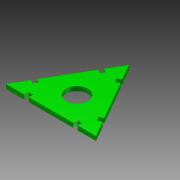
# Autodesk Inventor part: actuator
Saved by Autodesk Inventor 2012 (Build 160160000, 160)
## iProperties
Created: 2013-10-02
Part Number: actuator
Material: Default
Document SubType Name: Modeling
Designer: Nick
Density: 1 g/cm^3
Author: Nick
Autodesk Inventor part; units mm, degrees
ref_plane "YZ Plane" through (0, 0, 0) normal (1, 0, 0) x (0, 1, 0)
ref_plane "XZ Plane" through (0, 0, 0) normal (0, 1, 0) x (-1, 0, 0)
ref_plane "XY Plane" through (0, 0, 0) normal (0, 0, 1) x (1, 0, 0)
sketch "Sketch1" plane through (0, 0, 0) normal (0, 0, 1) x (1, 0, 0)
  circle A0 centre (0, 0) radius 7.5
  line L0 (31.1769, -18) -> (-31.1769, -18) construction
  line L1 (-31.1769, -18) -> (0, 36) construction
  line L2 (0, 36) -> (31.1769, -18) construction
  line L3 (15.5, -18) -> (15.5, -15)
  line L4 (15.5, -15) -> (18.5, -15)
  line L5 (18.5, -15) -> (18.5, -18)
  line L6 (-18.5, -18) -> (-18.5, -15)
  line L7 (-18.5, -15) -> (-15.5, -15)
  line L8 (-15.5, -15) -> (-15.5, -18)
  line L9 (-31.1769, -18) -> (15.5885, 9) construction
  line L10 (31.1769, -18) -> (-15.5885, 9) construction
  line L11 (0, 36) -> (0, -18) construction
  line L12 (6.3385, 25.0215) -> (3.7404, 23.5215)
  line L13 (3.7404, 23.5215) -> (5.2404, 20.9234)
  line L14 (5.2404, 20.9234) -> (7.8385, 22.4234)
  line L15 (23.3385, -4.4234) -> (20.7404, -5.9234)
  line L16 (20.7404, -5.9234) -> (22.2404, -8.5215)
  line L17 (22.2404, -8.5215) -> (24.8385, -7.0215)
  line L18 (-24.8385, -7.0215) -> (-22.2404, -8.5215)
  line L19 (-22.2404, -8.5215) -> (-20.7404, -5.9234)
  line L20 (-20.7404, -5.9234) -> (-23.3385, -4.4234)
  line L21 (-7.8385, 22.4234) -> (-5.2404, 20.9234)
  line L22 (-5.2404, 20.9234) -> (-3.7404, 23.5215)
  line L23 (-3.7404, 23.5215) -> (-6.3385, 25.0215)
  line L24 (-6.3385, 25.0215) -> (0, 36)
  line L25 (6.3385, 25.0215) -> (0, 36)
  line L26 (7.8385, 22.4234) -> (23.3385, -4.4234)
  line L27 (24.8385, -7.0215) -> (31.1769, -18)
  line L28 (31.1769, -18) -> (18.5, -18)
  line L29 (15.5, -18) -> (-15.5, -18)
  line L30 (-18.5, -18) -> (-31.1769, -18)
  line L31 (-31.1769, -18) -> (-24.8385, -7.0215)
  line L32 (-23.3385, -4.4234) -> (-7.8385, 22.4234)
  dimension "d3" = 15
  dimension "d4" = 18.5
  dimension "d5" = 18.5
  dimension "d8" = 3
  dimension "d9" = 18
  dimension "d10" = 3
  dimension "d11" = 3
  dimension "d12" = 18.5
  dimension "d13" = 3
  dimension "d14" = 3
  dimension "d15" = 18.5
  dimension "d16" = 3
  dimension "d17" = 3
  dimension "d18" = 18.5
  dimension "d19" = 3
  dimension "d20" = 3
  dimension "d21" = 3
  dimension "d22" = 18.5
  dimension "d23" = 3
  constraints: 66 end point, 14 perpendicular, 12 point on line, 7 collinear, 6 parallel, 3 midpoint, 2 coincident, 1 centre point, 1 horizontal, 7 other
  measures "d3" diameter of A0
  measures "d4" distance from line of L5 A0.centre
  measures "d5" horizontal distance of point (0, 0) L6.start
  measures "d8" distance between parallel lines of L0 L4
  measures "d9" distance from line of L0 point (0, 0)
  measures "d10" distance between parallel lines of L5 L3
  measures "d11" distance between parallel lines of L6 L8
  measures "d12" distance between parallel lines of L17 L9
  measures "d13" distance between parallel lines of L15 L17
  measures "d14" distance between parallel lines of L2 L16
  measures "d15" distance between parallel lines of L12 L9
  measures "d16" distance between parallel lines of L12 L14
  measures "d17" distance between parallel lines of L2 L13
  measures "d18" distance between parallel lines of L23 L10
  measures "d19" distance of L21.end L22.end
  measures "d20" distance between parallel lines of L1 L22
  measures "d21" distance of L19.end L20.end
  measures "d22" distance between parallel lines of L10 L18
  measures "d23" distance of L18.end L19.end
extrude "Extrusion2" add sketch "Sketch1" along normal blind 3
equation "\"d5\" = d4"
equation "\"d11\" = d10"
equation "\"d12\" = d4"
equation "\"d13\" = d10"
equation "\"d14\" = d8"
equation "\"d15\" = d4"
equation "\"d16\" = d13"
equation "\"d17\" = d8"
equation "\"d18\" = d4"
equation "\"d19\" = d10"
equation "\"d20\" = d8"
equation "\"d21\" = d8"
equation "\"d22\" = d4"
equation "\"d23\" = d10"
body "Solid2"
